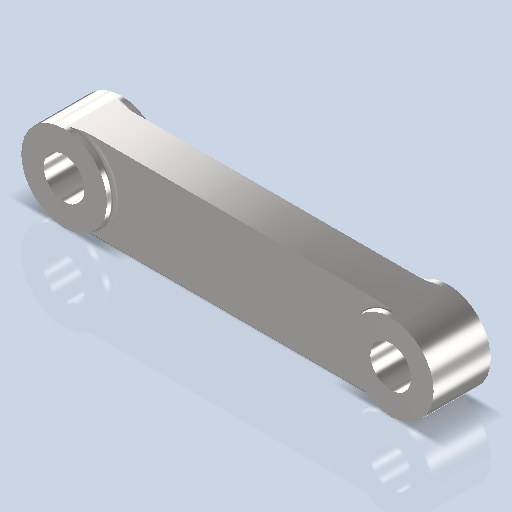
# Autodesk Inventor part: pleuel
Saved by Autodesk Inventor 2024 (Build 280153000, 153)
## iProperties
Created: 2024-04-30
Part Number: pleuel
Material: Edelstahl
Document SubType Name: Modeling
Designer: ffogue
Density: 8 g/cm^3
Appearance: Halbpoliert
Author: ffogue
Autodesk Inventor part; units mm, degrees
ref_plane "YZ Plane" through (0, 0, 0) normal (1, 0, 0) x (0, 1, 0)
ref_plane "XZ Plane" through (0, 0, 0) normal (0, 1, 0) x (-1, 0, 0)
ref_plane "XY Plane" through (0, 0, 0) normal (0, 0, 1) x (1, 0, 0)
sketch "Skizze1" plane through (0, 0, 0) normal (0, 1, 0) x (-1, 0, 0)
  line L0 (0, 5.25) -> (40, 5.25)
  line L1 (40, -5.25) -> (0, -5.25)
  line L2 (0, 0) -> (40, 0) construction
  circle A0 centre (0, 0) radius 5.25
  circle A1 centre (40, 0) radius 5.25
  dimension "d1" = 10.5
  dimension "d2" = 10.5
  dimension "d3" = 40
  constraints: 6 end point, 4 point on circle, 2 centre point, 2 horizontal, 1 coincident, 1 parallel, 1 point on line, 1 tangent, 1 vertical alignment, 1 other
  measures "d1" diameter of A0
  measures "d2" diameter of A1
  measures "d3" distance of L2.start L2.end
extrude "Extrusion1" add sketch "Skizze1" along normal mid plane 7 contours A0 | A1
extrude "Extrusion2" add sketch "Skizze1" along normal mid plane 5 contours L0 A1 L1 A0
sketch "Skizze2" plane through (-40, 3.5, 0) normal (0, 1, 0) x (1, 0, 0)
  circle A0 centre (0, 0) radius 5.25 projected
  point P0 (40, 0)
  constraints: 1 coincident
hole "Bohrung1" at (-40, 3.5, 0) direction (0, -1, 0) diameter 5 depth 7
hole "Bohrung2" at (0, 3.5, 0) direction (0, -1, 0) diameter 5 depth 7
fillet "Rundung1" radius 0.5 6 edges at (-34.75, 2.5, 0) (-34.75, -2.5, 0) (-3.7123, -2.5, -3.7123) (-3.7123, -2.5, 3.7123) (-3.7123, 2.5, 3.7123) (-3.7123, 2.5, -3.7123)
